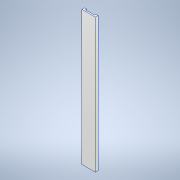
# Autodesk Inventor part: L_PlNKA800
Saved by Autodesk Inventor 2022 (Build 260153000, 153)
## iProperties
Created: 2023-08-15
Part Number: L_PlNKA800
Material: Aluminum 6061
Document SubType Name: Modeling
Designer: Kippi
Mass: 3564 g
Surface Area: 2626.4 cm^2
Volume: 1320 cm^3
Density: 2.7 g/cm^3
Appearance: Aluminum - Flat
Author: Kippi
Autodesk Inventor part; units mm, degrees
ref_plane "YZ Plane" through (0, 0, 0) normal (1, 0, 0) x (0, 1, 0)
ref_plane "XZ Plane" through (0, 0, 0) normal (0, 1, 0) x (-1, 0, 0)
ref_plane "XY Plane" through (0, 0, 0) normal (0, 0, 1) x (1, 0, 0)
sketch "Sketch1" plane through (0, 0, 0) normal (0, 1, 0) x (-1, 0, 0)
  line L0 (10, 10) -> (-90, 10)
  line L1 (-90, 10) -> (-90, -10)
  line L2 (-90, -10) -> (10, -10)
  line L3 (10, -10) -> (10, 10)
  line L4 (-6, -15) -> (-74, -15)
  line L5 (-74, -15) -> (-74, 0)
  line L6 (-74, 0) -> (-6, 0)
  line L7 (-6, 0) -> (-6, -15)
  point P0 (0, 0)
  point P1 (-74, -10)
  point P2 (-6, -10)
  dimension "d0" = 20
  dimension "d1" = 100
  dimension "d4" = 10
  dimension "d5" = 16
  dimension "d6" = 16
  constraints: 16 end point, 4 parallel, 2 horizontal, 2 perpendicular
  measures "d0" distance of L2.end L0.start
  measures "d1" distance of L1.end L2.end
  measures "d4" distance between parallel lines of L0 L6
  measures "d5" distance between parallel lines of L1 L5
  measures "d6" distance between parallel lines of L3 L7
extrude "Extrusion1" add sketch "Sketch1" along normal blind 1000 contours L3 L2 L7 L6 L5 L1 L0
body "Solid1"
